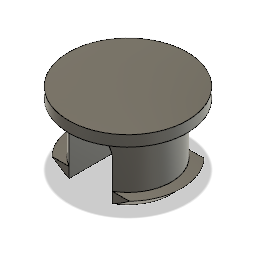
Clip (Autodesk Fusion 360 design; units mm, degrees)
Autodesk Fusion 360 part; units mm, degrees
sketch "Sketch2" plane through (0, 0, 0) normal (0, 1, 0) x (1, 0, 0)
  circle A0 centre (19.7031, -9.229) radius 4
  dimension "d6" = 8
  measures "d6" diameter of A0
extrude "Extrude2" add sketch "Sketch2" along normal blind 4.7
sketch "Sketch3" plane through (0, 4.7, 0) normal (0, 1, 0) x (-1, 0, 0)
  circle A0 centre (-19.7031, 9.229) radius 4
  circle A1 centre (-19.7031, 9.229) radius 5.5
  dimension "d9" = 11
  constraint concentric A0 A1
  measures "d9" diameter of A1
extrude "Extrude3" add sketch "Sketch3" along normal blind 1 contours A0 | A1
sketch "Sketch4" plane through (0, 0, 0) normal (0, -1, 0) x (1, 0, 0)
  circle A0 centre (19.7031, 9.229) radius 4
  circle A1 centre (19.7031, 9.229) radius 5
  dimension "d12" = 10
  constraint concentric A0 A1
  measures "d12" diameter of A1
extrude "Extrude4" add sketch "Sketch4" along normal blind 1 contours A0 | A1
chamfer "Chamfer1" distance 1 angle 45 1 edges at (15.0414, -1, 7.4209)
ref_plane "WorkPlane1" through (19.7031, 4.9209, 14.729) normal (0, 0, 1) x (-1, 0, 0)
sketch "Sketch5" plane through (19.7031, 4.7209, 14.729) normal (0, 0, 1) x (1, 0, 0)
  line L0 (-5, -4.7209) -> (5, -4.7209) construction
  line L1 (-2, 4.4802) -> (-2, -8.3463) construction
  line L2 (2, 4.6454) -> (2, -9.1996) construction
  line L3 (5.5, -0.0209) -> (-5.5, -0.0209)
  line L4 (-2, -5.7209) -> (2, -5.7209)
  line L5 (0, -0.0209) -> (0, -0.0209)
  line L6 (2, -2.0209) -> (2, -5.7209)
  line L7 (2, -5.7209) -> (-2, -5.7209)
  line L8 (-2, -5.7209) -> (-2, -2.0209)
  arc A0 (0, -0.0209) -> (-2, -2.0209) centre (0, -2.0209) ccw
  arc A1 (2, -2.0209) -> (0, -0.0209) centre (0, -2.0209) ccw
  dimension "d17" = 3
  dimension "d18" = 3
  dimension "d22" = 2
  dimension "d23" = 2
  constraint perpendicular L0 L1
  constraint vertical L2
  constraint coincident L1 L4.start
  constraint coincident L2 L4.end
  constraint perpendicular L2 L4
  constraint vertical L6
  constraint horizontal L7
  constraint vertical L8
  constraint tangent L8 A0
  constraint tangent L6 A1
  constraint coincident A0.centre A1.centre
  measures "d17" distance of L0.start L1
  measures "d18" distance of L0.end L2
  measures "d22" radius of A0
  measures "d23" radius of A1
extrude "Extrude6" cut sketch "Sketch5" against normal blind 13
sketch "Sketch6" plane through (0, 0, 0) normal (0, 1, 0) x (-1, 0, 0)
  line L0 (-17.7031, 5.7649) -> (-17.7031, 4.6464)
  arc A0 (-17.7031, 4.6464) -> (-17.7031, 13.8116) centre (-19.7031, 9.229) ccw
  line L1 (-17.7031, 13.8116) -> (-17.7031, 12.6931)
  arc A1 (-17.7031, 5.7649) -> (-17.7031, 12.6931) centre (-19.7031, 9.229) ccw
  line L2 (-13.4222, 12.6931) -> (-25.4959, 12.6931) construction
  line L3 (-25.6316, 5.7649) -> (-13.5986, 5.7649) construction
  line L4 (-14.1412, 3.3951) -> (-25.2924, 3.3951)
  line L5 (-25.2924, 3.3951) -> (-25.2924, 5.7649)
  line L6 (-25.2924, 5.7649) -> (-14.1412, 5.7649)
  line L7 (-14.1412, 5.7649) -> (-14.1412, 3.3951)
  line L8 (-13.7614, 12.6931) -> (-25.6316, 12.6931)
  line L9 (-25.6316, 12.6931) -> (-25.6316, 14.2478)
  line L10 (-25.6316, 14.2478) -> (-13.7614, 14.2478)
  line L11 (-13.7614, 14.2478) -> (-13.7614, 12.6931)
  constraint horizontal L2
  constraint parallel L2 L3
  constraint horizontal L4
  constraint vertical L5
  constraint horizontal L6
  constraint vertical L7
  constraint coincident L3 L5.end
  constraint horizontal L8
  constraint vertical L9
  constraint horizontal L10
  constraint vertical L11
  constraint coincident L2 L8.start
extrude "Extrude7" cut sketch "Sketch6" against normal blind 3 contours L0 A0 L6 | L0 A0 L4 L5 L6 L7 | A0 L1 L8 L9 L10 L11 | A0 L1 L8
